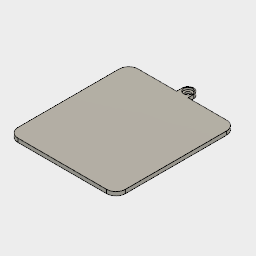
CaseV2 Back Cover v4 (Autodesk Fusion 360 design; units mm, degrees)
Autodesk Fusion 360 part; units mm, degrees
note: some values were not read from the file. Set by a fixed rule: which face or edge a step refers to.
sketch "Sketch1" plane through (0, 0, 0) normal (0, 1, 0) x (1, 0, 0)
  line L0 (28.4985, -31.7) -> (-28.4985, -31.7)
  line L1 (-28.4985, -31.7) -> (-28.4985, 31.7)
  line L2 (-28.4985, 31.7) -> (28.4985, 31.7)
  line L3 (28.4985, 31.7) -> (28.4985, -31.7)
  line L4 (28.4985, -31.7) -> (-28.4985, 31.7) construction
  line L5 (-28.4985, -31.7) -> (28.4985, 31.7) construction
  line L6 (3, 31.7) -> (-3, 31.7)
  line L7 (-3, 31.7) -> (-3, 34.7)
  line L8 (-3, 34.7) -> (3, 34.7)
  line L9 (3, 34.7) -> (3, 31.7)
  line L10 (3, 31.7) -> (-3, 34.7) construction
  line L11 (-3, 31.7) -> (3, 34.7) construction
  arc A0 (3, 34.7) -> (-3, 34.7) centre (0, 34.7) ccw
  circle A1 centre (0, 34.7) radius 1.25
  point P0 (0, 33.2)
  dimension "d1" = 56.997
  dimension "d2" = 63.4
  dimension "d3" = 6
  dimension "d4" = 3
  dimension "d5" = 2.5
  measures "d1" distance of L1.end L2.end
  measures "d2" distance of L0.end L1.end
  measures "d3" distance of L7.end L8.end
  measures "d4" distance of L6.end L7.end
  measures "d5" diameter of A1
extrude "Extrude1" add sketch "Sketch1" along normal blind 2 contours L0 L1 L2 L3 L6 | L2 L6 L7 L8 L9 A1 | L8 A0 A1
sketch "Sketch2" plane through (0, 2, 0) normal (0, 1, 0) x (-1, 0, 0)
  circle A0 centre (0, -34.7) radius 1.25
  line L0 (-3, -31.7) -> (-3, -34.7)
  arc A1 (-3, -34.7) -> (3, -34.7) centre (0, -34.7) ccw
  line L1 (3, -34.7) -> (3, -31.7)
  line L2 (3, -31.7) -> (28.4985, -31.7)
  line L3 (28.4985, -31.7) -> (28.4985, 31.7)
  line L4 (28.4985, 31.7) -> (-28.4985, 31.7)
  line L5 (-28.4985, 31.7) -> (-28.4985, -31.7)
  line L6 (-28.4985, -31.7) -> (-3, -31.7)
  circle A2 centre (0, -34.7) radius 2.4
  dimension "d8" = 4.8
  measures "d8" diameter of A2
extrude "Extrude2" cut sketch "Sketch2" against normal blind 1.4 contours A2
extrude "Extrude3" add 1 faces at (-2.0077, 0.6, -34.8192) along direction (0, 1, 0) blind 0.4
fillet "Fillet1" chord length 7 4 edges at (-28.4985, 1, -31.7) (28.4985, 1, -31.7) (28.4985, 1, 31.7) (-28.4985, 1, 31.7)
move_face "OffsetFaces1" offset -0.25 1 faces at (-28.4985, 0.6667, 8.9168)
move_face "OffsetFaces2" offset -0.25 1 faces at (28.4985, 1.3333, 8.9168)
move_face "OffsetFaces3" offset -0.25 1 faces at (7.7663, 0.6667, 31.7)
